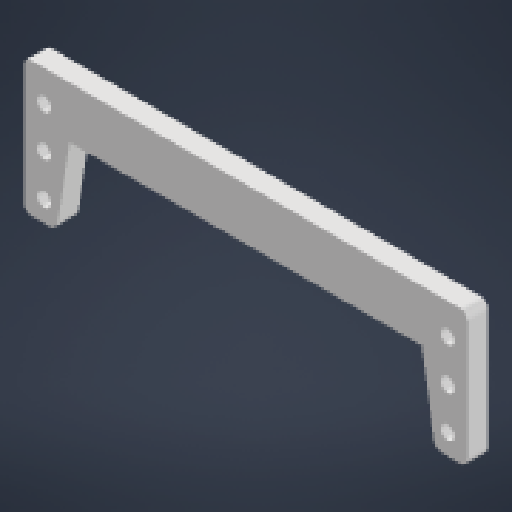
# Autodesk Inventor part: parkbrake
Saved by Autodesk Inventor 2025.2 (Build 292293000, 293)
## iProperties
Created: 2026-01-05
Part Number: parkbrake
Material: Acetal Resin, Black
Document SubType Name: Modeling
Designer: cloudy
Density: 1.425 g/cm^3
Appearance: Smooth - Black
Author: cloudy
Autodesk Inventor part; units mm, degrees
ref_plane "YZ Plane" through (0, 0, 0) normal (1, 0, 0) x (0, 1, 0)
ref_plane "XZ Plane" through (0, 0, 0) normal (0, 1, 0) x (-1, 0, 0)
ref_plane "XY Plane" through (0, 0, 0) normal (0, 0, 1) x (1, 0, 0)
sketch "Sketch1" plane through (0, 0, 0) normal (0, 0, 1) x (1, 0, 0)
  circle A0 centre (12.7, 38.1) radius 2.1844 projected
  circle A1 centre (-111.125, 38.1) radius 2.1844 projected
  circle A2 centre (-111.125, 25.4) radius 2.1844 projected
  circle A3 centre (12.7, 25.4) radius 2.1844 projected
  line L0 (-117.475, 45.085) -> (-117.475, 8.89)
  line L1 (-114.935, 6.35) -> (-109.4756, 6.35)
  line L2 (-106.9685, 8.4826) -> (-103.1875, 31.75)
  line L3 (-103.1875, 31.75) -> (4.7625, 31.75)
  line L4 (4.7625, 31.75) -> (8.5435, 8.4826)
  line L5 (11.0506, 6.35) -> (16.51, 6.35)
  line L6 (19.05, 8.89) -> (19.05, 45.085)
  line L7 (16.51, 47.625) -> (-114.935, 47.625)
  line L8 (-49.2125, 31.75) -> (-49.2125, 47.625) construction
  arc A4 (-114.935, 47.625) -> (-117.475, 45.085) centre (-114.935, 45.085) ccw
  arc A5 (-117.475, 8.89) -> (-114.935, 6.35) centre (-114.935, 8.89) ccw
  arc A6 (16.51, 6.35) -> (19.05, 8.89) centre (16.51, 8.89) ccw
  arc A7 (19.05, 45.085) -> (16.51, 47.625) centre (16.51, 45.085) ccw
  arc A8 (-109.4756, 6.35) -> (-106.9685, 8.4826) centre (-109.4756, 8.89) ccw
  arc A9 (8.5435, 8.4826) -> (11.0506, 6.35) centre (11.0506, 8.89) ccw
  circle A10 centre (-111.125, 12.7) radius 2.1844 projected
  circle A11 centre (12.7, 12.7) radius 2.1844 projected
  point P0 (0, 0)
  point P1 (8.89, 6.35)
  point P2 (19.05, 6.35)
  dimension "d0" = 6.35
  dimension "d1" = 6.35
  dimension "d2" = 9.525
  dimension "d4" = 15.875
  dimension "d5" = 107.95
  dimension "d6" = 10.16
  dimension "d7" = 2.54
  dimension "d8" = 2.54
  dimension "d9" = 2.54
  dimension "d12" = 6.35
  constraints: 18 end point, 12 point on circle, 12 tangent, 6 centre point, 6 point on line, 3 equal radius, 3 vertical, 2 horizontal, 2 midpoint, 2 perpendicular, 1 equal length
  measures "d0" distance from line of L6 A0.centre
  measures "d1" distance from line of L0 A1.centre
  measures "d2" distance from line of L7 A0.centre
  measures "d4" distance between parallel lines of L7 L3
  measures "d5" distance of L2.end L3.end
  measures "d6" distance of point (8.89, 6.35) point (19.05, 6.35)
  measures "d7" radius of A4
  measures "d8" radius of A8
  measures "d9" radius of A9
  measures "d12" distance from line of A11.centre L5
extrude "Extrusion1" add sketch "Sketch1" along normal blind 6.35
equation "\"d0\" = d1"
equation "\"d10\" = d1"
body "Solid1"
